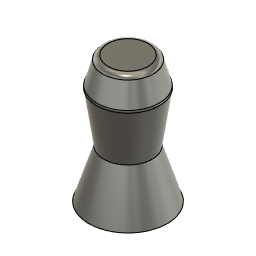
forme3proto v3 (Autodesk Fusion 360 design; units mm, degrees)
Autodesk Fusion 360 part; units mm, degrees
sketch "Esquisse1" plane through (0, 0, 0) normal (0, 0, 1) x (1, 0, 0)
  line L0 (0, 0) -> (-65, 0)
  line L1 (-65, 0) -> (-40, 80)
  line L2 (-40, 80) -> (-52.5, 165)
  line L3 (-52.5, 165) -> (-40, 210)
  line L4 (-40, 210) -> (0, 210)
  line L5 (0, 210) -> (0, 0)
  dimension "d1" = 65
  dimension "d3" = 45
  dimension "d4" = 85
  dimension "d5" = 80
  dimension "d6" = 40
  dimension "d7" = 52.5
  dimension "d8" = 40
  constraint coincident L0.start L5.end
  constraint horizontal L0
  constraint horizontal L4
  constraint perpendicular L0 L5
  measures "d1" distance of L0.start L0.end
  measures "d3" vertical distance of L2.end L3.end
  measures "d4" vertical distance of L1.end L2.end
  measures "d5" vertical distance of L0.end L1.end
  measures "d6" distance of L1.end L5
  measures "d7" distance of L2.end L5
  measures "d8" distance of L3.end L4.end
revolve "Révolution1" add sketch "Esquisse1" angle 360 about axis through (0, 210, 0) along (0, -1, 0)
fillet "Congé1" radius 9 1 edges at (-48.9472, 165, 18.9848)
fillet "Congé2" radius 9 1 edges at (-37.2931, 210, 14.4646)
shell "Coque1" thickness 2 removed faces 1 at (20.2416, 0, -0.2148)
